Autodesk Inventor part; units mm, degrees
(part 4 of 4)
sketch "Sketch11" plane through (0, 10, 0) normal (0, 1, 0) x (1, 0, 0)
  line L0 (-6.9956, -98.5274) -> (-7.1309, -98.4307) construction
  line L1 (97.89, -8.7381) -> (95.2599, -7.1233) construction
  line L2 (96.5749, -9.4923) -> (97.861, -10.2466) construction
  line L3 (92.9585, -8.419) -> (92.2333, -8.0129) construction
  line L4 (92.5717, -7.1523) -> (92.6491, -7.278) construction
  line L5 (92.6491, -7.278) -> (95.2115, -8.7188) construction
  line L6 (95.724, -6.4464) -> (97.861, -7.7131) construction
  circle A0 centre (0, -95) radius 2 construction
  circle A1 centre (95, 0) radius 2 construction
  line L7 (34.0692, -36.9904) -> (16.7487, -26.9904) construction
  arc A2 (16.7487, -26.9904) -> (16.0167, -24.2583) centre (15.0167, -25.9904) ccw construction
  line L8 (16.0167, -24.2583) -> (29.0167, -1.7417) construction
  arc A3 (29.0167, -1.7417) -> (31.7487, -1.0096) centre (30.0167, -0.0096) ccw construction
  line L9 (31.7487, -1.0096) -> (49.0692, -11.0096) construction
  arc A4 (49.0692, -11.0096) -> (49.8013, -13.7417) centre (50.8013, -12.0096) ccw construction
  line L10 (49.8013, -13.7417) -> (36.8013, -36.2583) construction
  arc A5 (36.8013, -36.2583) -> (34.0692, -36.9904) centre (35.8013, -37.9904) ccw construction
  line L11 (16.0167, -27.7224) -> (33.8013, -37.9904) construction
  arc A6 (33.8013, -37.9904) -> (37.5333, -36.9904) centre (35.8013, -37.9904) ccw construction
  line L12 (37.5333, -36.9904) -> (50.8013, -14.0096) construction
  arc A7 (50.8013, -14.0096) -> (49.8013, -10.2776) centre (50.8013, -12.0096) ccw construction
  line L13 (49.8013, -10.2776) -> (32.0167, -0.0096) construction
  arc A8 (32.0167, -0.0096) -> (28.2846, -1.0096) centre (30.0167, -0.0096) ccw construction
  line L14 (28.2846, -1.0096) -> (15.0167, -23.9904) construction
  arc A9 (15.0167, -23.9904) -> (16.0167, -27.7224) centre (15.0167, -25.9904) ccw construction
  line L15 (-49.0692, -11.0096) -> (-31.7487, -1.0096) construction
  arc A10 (-31.7487, -1.0096) -> (-29.0167, -1.7417) centre (-30.0167, -0.0096) ccw construction
  line L16 (-29.0167, -1.7417) -> (-16.0167, -24.2583) construction
  arc A11 (-16.0167, -24.2583) -> (-16.7487, -26.9904) centre (-15.0167, -25.9904) ccw construction
  line L17 (-16.7487, -26.9904) -> (-34.0692, -36.9904) construction
  arc A12 (-34.0692, -36.9904) -> (-36.8013, -36.2583) centre (-35.8013, -37.9904) ccw construction
  line L18 (-36.8013, -36.2583) -> (-49.8013, -13.7417) construction
  arc A13 (-49.8013, -13.7417) -> (-49.0692, -11.0096) centre (-50.8013, -12.0096) ccw construction
  line L19 (-32.0167, -0.0096) -> (-49.8013, -10.2776) construction
  arc A14 (-49.8013, -10.2776) -> (-50.8013, -14.0096) centre (-50.8013, -12.0096) ccw construction
  line L20 (-50.8013, -14.0096) -> (-37.5333, -36.9904) construction
  arc A15 (-37.5333, -36.9904) -> (-33.8013, -37.9904) centre (-35.8013, -37.9904) ccw construction
  line L21 (-33.8013, -37.9904) -> (-16.0167, -27.7224) construction
  arc A16 (-16.0167, -27.7224) -> (-15.0167, -23.9904) centre (-15.0167, -25.9904) ccw construction
  line L22 (-15.0167, -23.9904) -> (-28.2846, -1.0096) construction
  arc A17 (-28.2846, -1.0096) -> (-32.0167, -0.0096) centre (-30.0167, -0.0096) ccw construction
  line L23 (-46.6246, 31.9097) -> (-46.6246, 8.9097) construction
  line L24 (-46.6246, 8.9097) -> (-69.6246, 8.9097) construction
  line L25 (-69.6246, 8.9097) -> (-69.6246, 31.9097) construction
  line L26 (-69.6246, 31.9097) -> (-46.6246, 31.9097) construction
  line L27 (-45.6246, 7.9097) -> (-45.6246, 32.9097) construction
  line L28 (-45.6246, 32.9097) -> (-70.6246, 32.9097) construction
  line L29 (-70.6246, 32.9097) -> (-70.6246, 7.9097) construction
  line L30 (-70.6246, 7.9097) -> (-45.6246, 7.9097) construction
  line L31 (-23.9006, 30.2452) -> (-23.9006, 7.7452) construction
  line L32 (-23.9006, 7.7452) -> (-41.9006, 7.7452) construction
  line L33 (-41.9006, 7.7452) -> (-41.9006, 30.2452) construction
  line L34 (-41.9006, 30.2452) -> (-23.9006, 30.2452) construction
  line L35 (-32.1006, 6.7452) -> (-22.9006, 6.7452) construction
  line L36 (-22.9006, 6.7452) -> (-22.9006, 31.2452) construction
  line L37 (-22.9006, 31.2452) -> (-32.1006, 31.2452) construction
  arc A18 (-32.1006, 31.2452) -> (-33.7006, 31.2452) centre (-32.9006, 31.2452) ccw construction
  line L38 (-33.7006, 31.2452) -> (-42.9006, 31.2452) construction
  line L39 (-42.9006, 31.2452) -> (-42.9006, 6.7452) construction
  line L40 (-42.9006, 6.7452) -> (-33.7006, 6.7452) construction
  arc A19 (-33.7006, 6.7452) -> (-32.1006, 6.7452) centre (-32.9006, 6.7452) ccw construction
  line L41 (15, 48) -> (15, 28) construction
  arc A20 (15, 28) -> (13, 26) centre (15, 26) ccw construction
  line L42 (13, 26) -> (-13, 26) construction
  arc A21 (-13, 26) -> (-15, 28) centre (-15, 26) ccw construction
  line L43 (-15, 28) -> (-15, 48) construction
  arc A22 (-15, 48) -> (-13, 50) centre (-15, 50) ccw construction
  line L44 (-13, 50) -> (13, 50) construction
  arc A23 (13, 50) -> (15, 48) centre (15, 50) ccw construction
  line L45 (16, 27.7321) -> (16, 48.2679) construction
  arc A24 (16, 48.2679) -> (13.2679, 51) centre (15, 50) ccw construction
  line L46 (13.2679, 51) -> (-13.2679, 51) construction
  arc A25 (-13.2679, 51) -> (-16, 48.2679) centre (-15, 50) ccw construction
  line L47 (-16, 48.2679) -> (-16, 27.7321) construction
  arc A26 (-16, 27.7321) -> (-13.2679, 25) centre (-15, 26) ccw construction
  line L48 (-13.2679, 25) -> (13.2679, 25) construction
  arc A27 (13.2679, 25) -> (16, 27.7321) centre (15, 26) ccw construction
  line L49 (38.8707, 50.1548) -> (54.6756, 59.2798) construction
  line L50 (54.6756, 59.2798) -> (78.6756, 17.7106) construction
  line L51 (78.6756, 17.7106) -> (62.8707, 8.5856) construction
  arc A28 (62.8707, 8.5856) -> (61.5716, 7.8356) centre (62.7211, 7.3446) ccw construction
  line L52 (61.5716, 7.8356) -> (45.7667, -1.2894) construction
  line L53 (45.7667, -1.2894) -> (21.7667, 40.2798) construction
  line L54 (21.7667, 40.2798) -> (37.5716, 49.4048) construction
  arc A29 (37.5716, 49.4048) -> (38.8707, 50.1548) centre (37.7211, 50.6458) ccw construction
  line L55 (63.8037, 7.9696) -> (80.0417, 17.3446) construction
  line L56 (80.0417, 17.3446) -> (55.0417, 60.6458) construction
  line L57 (55.0417, 60.6458) -> (38.8037, 51.2708) construction
  arc A30 (38.8037, 51.2708) -> (36.6386, 50.0208) centre (37.7211, 50.6458) ccw construction
  line L58 (36.6386, 50.0208) -> (20.4006, 40.6458) construction
  line L59 (20.4006, 40.6458) -> (45.4006, -2.6554) construction
  line L60 (45.4006, -2.6554) -> (61.6386, 6.7196) construction
  arc A31 (61.6386, 6.7196) -> (63.8037, 7.9696) centre (62.7211, 7.3446) ccw construction
  line L61 (28, -43) -> (28, -89) construction
  line L62 (28, -89) -> (-28, -89) construction
  line L63 (-28, -89) -> (-28, -43) construction
  line L64 (-28, -43) -> (-8, -43) construction
  line L65 (-8, -43) -> (-8, -43.9952) construction
  line L66 (-8, -43.9952) -> (8, -43.9952) construction
  line L67 (8, -43.9952) -> (8, -43) construction
  line L68 (8, -43) -> (28, -43) construction
  line L69 (-27.75, -90) -> (27.75, -90) construction
  arc A32 (27.75, -90) -> (29, -88.75) centre (29, -90) ccw construction
  line L70 (29, -88.75) -> (29, -43.25) construction
  arc A33 (29, -43.25) -> (27.75, -42) centre (29, -42) ccw construction
  line L71 (27.75, -42) -> (8, -42) construction
  line L72 (8, -42) -> (8, -23.9952) construction
  line L73 (8, -23.9952) -> (-8, -23.9952) construction
  line L74 (-8, -23.9952) -> (-8, -42) construction
  line L75 (-8, -42) -> (-27.75, -42) construction
  arc A34 (-27.75, -42) -> (-29, -43.25) centre (-29, -42) ccw construction
  line L76 (-29, -43.25) -> (-29, -88.75) construction
  arc A35 (-29, -88.75) -> (-27.75, -90) centre (-29, -90) ccw construction
  line L77 (0.5057, 40.2674) -> (2.684, 40.2674) construction
  line L78 (2.684, 40.2674) -> (2.684, 41.3663) construction
  line L79 (0.2042, 43.0389) -> (-1.0405, 43.0389) construction
  line L80 (-1.0405, 43.0389) -> (-1.0405, 32.2253) construction
  line L81 (-1.0405, 32.2253) -> (-3.1702, 32.2253) construction
  line L82 (-3.1702, 32.2253) -> (-3.1702, 31) construction
  line L83 (-3.1702, 31) -> (2.684, 31) construction
  line L84 (2.684, 31) -> (2.684, 32.2253) construction
  line L85 (2.684, 32.2253) -> (0.5057, 32.2253) construction
  line L86 (0.5057, 32.2253) -> (0.5057, 40.2674) construction
  line L87 (11.4709, -68.4771) -> (10.6948, -68.4771) construction
  line L88 (10.6948, -68.4771) -> (10.6948, -69.1) construction
  line L89 (10.6948, -69.1) -> (13.0577, -69.1) construction
  line L90 (13.0577, -69.1) -> (13.0577, -68.4771) construction
  line L91 (13.0577, -68.4771) -> (12.2816, -68.4771) construction
  line L92 (12.2816, -68.4771) -> (12.2816, -63.6229) construction
  line L93 (12.2816, -63.6229) -> (13.0577, -63.6229) construction
  line L94 (13.0577, -63.6229) -> (13.0577, -63) construction
  line L95 (13.0577, -63) -> (10.6948, -63) construction
  line L96 (10.6948, -63) -> (10.6948, -63.6229) construction
  line L97 (10.6948, -63.6229) -> (11.4709, -63.6229) construction
  line L98 (11.4709, -63.6229) -> (11.4709, -68.4771) construction
  line L99 (17.4473, -69.1) -> (17.4473, -63) construction
  line L100 (17.4473, -63) -> (16.6366, -63) construction
  line L101 (16.6366, -63) -> (16.6366, -65.2739) construction
  line L102 (16.6366, -65.2739) -> (15.9495, -65.2739) construction
  line L103 (15.9149, -69.1) -> (17.4473, -69.1) construction
  line L104 (16.0829, -65.966) -> (16.6366, -65.966) construction
  line L105 (16.6366, -65.966) -> (16.6366, -68.3981) construction
  line L106 (16.6366, -68.3981) -> (15.9643, -68.3981) construction
  line L107 (-5.2028, -67.8444) -> (-5.2621, -67.8444) construction
  line L108 (-5.2621, -67.8444) -> (-5.2621, -68.8133) construction
  line L109 (-1.4113, -64.3841) -> (-1.352, -64.3841) construction
  line L110 (-1.352, -64.3841) -> (-1.352, -63.3658) construction
  line L111 (21.0806, -69.1) -> (22.6526, -69.1) construction
  line L112 (22.6526, -69.1) -> (22.6526, -63) construction
  line L113 (22.6526, -63) -> (21.8419, -63) construction
  line L114 (21.8419, -63) -> (21.8419, -65.4271) construction
  line L115 (21.8419, -65.4271) -> (20.9125, -65.4271) construction
  line L116 (20.9125, -65.4271) -> (18.9846, -63) construction
  line L117 (18.9846, -63) -> (17.9317, -63) construction
  line L118 (17.9317, -63) -> (20.1018, -65.6545) construction
  line L119 (21.13, -66.1044) -> (21.8419, -66.1044) construction
  line L120 (21.8419, -66.1044) -> (21.8419, -68.3981) construction
  line L121 (21.8419, -68.3981) -> (21.0361, -68.3981) construction
  line L122 (-10.9568, -63) -> (-11.7279, -63) construction
  line L123 (-11.7279, -63) -> (-11.7279, -67.5775) construction
  line L124 (-11.7279, -67.5775) -> (-10.9568, -67.5775) construction
  line L125 (-10.9568, -67.5775) -> (-10.9568, -63) construction
  line L126 (-15.7419, -65.7979) -> (-13.3246, -65.7979) construction
  line L127 (-13.3246, -65.2096) -> (-16.4932, -65.2096) construction
  line L128 (-16.4932, -65.2096) -> (-16.4932, -65.6298) construction
  line L129 (-16.4092, -63.2818) -> (-16.4092, -64.1221) construction
  line L130 (-16.4092, -64.1221) -> (-16.3647, -64.1221) construction
  line L131 (4.9754, -68.0669) -> (4.9754, -66.0006) construction
  line L132 (4.9754, -66.0006) -> (7.0417, -66.0006) construction
  line L133 (7.0417, -66.0006) -> (7.0417, -65.3431) construction
  line L134 (7.0417, -65.3431) -> (4.9754, -65.3431) construction
  line L135 (4.9754, -65.3431) -> (4.9754, -63.2768) construction
  line L136 (4.9754, -63.2768) -> (4.2932, -63.2768) construction
  line L137 (4.2932, -63.2768) -> (4.2932, -65.3431) construction
  line L138 (4.2932, -65.3431) -> (2.2269, -65.3431) construction
  line L139 (2.2269, -65.3431) -> (2.2269, -66.0006) construction
  line L140 (2.2269, -66.0006) -> (4.2932, -66.0006) construction
  line L141 (4.2932, -66.0006) -> (4.2932, -68.0669) construction
  line L142 (4.2932, -68.0669) -> (4.9754, -68.0669) construction
  line L143 (-17.2891, -63) -> (-18.0603, -63) construction
  line L144 (-18.0603, -63) -> (-18.0603, -69.3719) construction
  line L145 (-18.0603, -69.3719) -> (-17.2891, -69.3719) construction
  line L146 (-17.2891, -69.3719) -> (-17.2891, -63) construction
  line L147 (-6.2656, -69.3719) -> (-6.2656, -63) construction
  line L148 (-6.2656, -63) -> (-7.0368, -63) construction
  line L149 (-7.0368, -63) -> (-7.0368, -66.4207) construction
  line L150 (-9.0882, -65.61) -> (-9.0882, -63) construction
  line L151 (-9.0882, -63) -> (-9.8594, -63) construction
  line L152 (-9.8594, -63) -> (-9.8594, -65.9709) construction
  line L153 (-7.0368, -67.0683) -> (-7.0368, -69.3719) construction
  line L154 (-7.0368, -69.3719) -> (-6.2656, -69.3719) construction
  line L155 (-34.4486, 9.7771) -> (-34.4486, 9.2238) construction
  line L156 (-34.4486, 9.2238) -> (-31.4006, 9.2238) construction
  line L157 (-31.4006, 9.2238) -> (-31.4006, 9.6017) construction
  line L158 (-31.4006, 9.6017) -> (-34.0263, 9.6017) construction
  line L159 (-34.0263, 9.6017) -> (-32.2404, 10.3897) construction
  line L160 (-32.2404, 10.3897) -> (-32.2404, 10.6367) construction
  line L161 (-32.2404, 10.6367) -> (-34.0263, 11.432) construction
  line L162 (-34.0263, 11.432) -> (-31.4006, 11.432) construction
  line L163 (-31.4006, 11.432) -> (-31.4006, 11.8371) construction
  line L164 (-31.4006, 11.8371) -> (-34.4486, 11.8371) construction
  line L165 (-34.4486, 11.8371) -> (-34.4486, 11.2739) construction
  line L166 (-34.4486, 11.2739) -> (-32.7517, 10.5379) construction
  line L167 (-32.7517, 10.5379) -> (-34.4486, 9.7771) construction
  line L168 (-11.7823, -68.3387) -> (-11.7823, -69.1395) construction
  line L169 (-11.7823, -69.1395) -> (-10.9073, -69.1395) construction
  line L170 (-10.9073, -69.1395) -> (-10.9073, -68.3387) construction
  line L171 (-10.9073, -68.3387) -> (-11.7823, -68.3387) construction
  line L172 (-31.4006, 14.769) -> (-31.4006, 15.1543) construction
  line L173 (-31.4006, 15.1543) -> (-34.5845, 15.1543) construction
  line L174 (-34.5845, 15.1543) -> (-34.5845, 14.769) construction
  line L175 (-34.5845, 14.769) -> (-31.4006, 14.769) construction
  line L176 (-21.9407, -63.4647) -> (-21.9407, -63) construction
  line L177 (-21.9407, -63) -> (-22.7119, -63) construction
  line L178 (-22.7119, -63) -> (-22.7119, -69.3719) construction
  line L179 (-22.7119, -69.3719) -> (-21.9407, -69.3719) construction
  line L180 (-21.9407, -69.3719) -> (-21.9407, -67.3946) construction
  line L181 (-21.9407, -66.7569) -> (-21.9407, -64.1122) construction
  line L182 (-31.4006, 17.1303) -> (-31.4006, 17.5157) construction
  line L183 (-31.4006, 17.5157) -> (-33.6879, 17.5157) construction
  line L184 (-33.6879, 17.5157) -> (-33.6879, 17.1303) construction
  line L185 (-33.6879, 17.1303) -> (-31.4006, 17.1303) construction
  line L186 (-35.1477, -24.1889) -> (-33.6654, -23.3332) construction
  line L187 (-33.6654, -23.3332) -> (-33.7092, -23.2574) construction
  line L188 (-26.507, -19.4922) -> (-25.0332, -18.6413) construction
  line L189 (-25.0332, -18.6413) -> (-28.7333, -12.2324) construction
  line L190 (-28.7333, -12.2324) -> (-29.9376, -12.9277) construction
  line L191 (-29.9376, -12.9277) -> (-26.9911, -18.0312) construction
  line L192 (-31.8279, 18.4666) -> (-33.1272, 18.4666) construction
  line L193 (-33.4483, 18.4666) -> (-33.6879, 18.4666) construction
  line L194 (-33.6879, 18.4666) -> (-33.6879, 18.0813) construction
  line L195 (-33.6879, 18.0813) -> (-30.5584, 18.0813) construction
  line L196 (-30.5584, 18.0813) -> (-30.5584, 18.4666) construction
  line L197 (-30.5584, 18.4666) -> (-31.5167, 18.4666) construction
  line L198 (-32.3837, 12.793) -> (-33.6879, 12.793) construction
  line L199 (-33.6879, 12.793) -> (-33.6879, 12.4077) construction
  line L200 (-33.6879, 12.4077) -> (-32.2034, 12.4077) construction
  line L201 (-31.6526, 13.818) -> (-31.4006, 13.818) construction
  line L202 (-31.4006, 13.818) -> (-31.4006, 14.2034) construction
  line L203 (-31.4006, 14.2034) -> (-33.6879, 14.2034) construction
  line L204 (-33.6879, 14.2034) -> (-33.6879, 13.818) construction
  line L205 (-33.6879, 13.818) -> (-31.9786, 13.818) construction
  line L206 (-31.4006, 20.4056) -> (-31.4006, 20.7909) construction
  line L207 (-31.4006, 20.7909) -> (-34.5845, 20.7909) construction
  line L208 (-34.5845, 20.7909) -> (-34.5845, 20.4056) construction
  line L209 (-34.5845, 20.4056) -> (-31.4006, 20.4056) construction
  line L210 (-33.3692, 16.13) -> (-33.3692, 16.8389) construction
  line L211 (-33.3692, 16.8389) -> (-33.6879, 16.8389) construction
  line L212 (-33.6879, 16.8389) -> (-33.6879, 16.13) construction
  line L213 (-33.6879, 16.13) -> (-34.3449, 16.13) construction
  line L214 (-34.3449, 16.13) -> (-34.3449, 15.7446) construction
  line L215 (-34.3449, 15.7446) -> (-33.6879, 15.7446) construction
  line L216 (-33.6879, 15.7446) -> (-33.6879, 15.4853) construction
  line L217 (-33.6879, 15.4853) -> (-33.3692, 15.4853) construction
  line L218 (-33.3692, 15.4853) -> (-33.3692, 15.7446) construction
  line L219 (-33.3692, 15.7446) -> (-32.1021, 15.7446) construction
  line L220 (-31.4204, 16.8389) -> (-31.7662, 16.8389) construction
  line L221 (-31.7662, 16.8389) -> (-31.7662, 16.8166) construction
  line L222 (-32.28, 16.13) -> (-33.3692, 16.13) construction
  line L223 (-32.7987, 27.0771) -> (-32.7987, 25.8692) construction
  line L224 (-32.5047, 25.8692) -> (-32.5047, 27.4525) construction
  line L225 (-32.5047, 27.4525) -> (-32.7147, 27.4525) construction
  line L226 (-31.5414, 27.4105) -> (-31.9613, 27.4105) construction
  line L227 (-31.9613, 27.4105) -> (-31.9613, 27.3883) construction
  line L228 (-34.0683, 17.5428) -> (-34.4684, 17.5428) construction
  line L229 (-34.4684, 17.5428) -> (-34.4684, 17.1056) construction
  line L230 (-34.4684, 17.1056) -> (-34.0683, 17.1056) construction
  line L231 (-34.0683, 17.1056) -> (-34.0683, 17.5428) construction
  line L232 (-33.347, 28.2281) -> (-33.6879, 28.2281) construction
  line L233 (-33.6879, 28.2281) -> (-33.6879, 27.8428) construction
  line L234 (-33.6879, 27.8428) -> (-31.4006, 27.8428) construction
  line L235 (-31.4006, 27.8428) -> (-31.4006, 28.2281) construction
  line L236 (-31.4006, 28.2281) -> (-33.0234, 28.2281) construction
  line L237 (-33.2754, 29.0358) -> (-33.2754, 29.0556) construction
  line L238 (-33.2754, 29.0556) -> (-33.6755, 29.0556) construction
  line L239 (-32.5047, 21.5887) -> (-32.5047, 23.172) construction
  line L240 (-32.5047, 23.172) -> (-32.7147, 23.172) construction
  line L241 (-31.5414, 23.13) -> (-31.9613, 23.13) construction
  line L242 (-31.9613, 23.13) -> (-31.9613, 23.1078) construction
  line L243 (-32.7987, 22.7965) -> (-32.7987, 21.5887) construction
  line L244 (-32.8357, 24.3354) -> (-33.6879, 23.7821) construction
  line L245 (-33.6879, 23.7821) -> (-33.6879, 23.3103) construction
  line L246 (-33.6879, 23.3103) -> (-32.5344, 24.0958) construction
  line L247 (-32.5344, 24.0958) -> (-31.4006, 23.3029) construction
  line L248 (-31.4006, 23.3029) -> (-31.4006, 23.7401) construction
  line L249 (-31.4006, 23.7401) -> (-32.2602, 24.3107) construction
  line L250 (-32.2602, 24.3107) -> (-31.4006, 24.8664) construction
  line L251 (-31.4006, 24.8664) -> (-31.4006, 25.3382) construction
  line L252 (-31.4006, 25.3382) -> (-32.5591, 24.5503) construction
  line L253 (-32.5591, 24.5503) -> (-33.6879, 25.3382) construction
  line L254 (-33.6879, 25.3382) -> (-33.6879, 24.901) construction
  line L255 (-33.6879, 24.901) -> (-32.8357, 24.3354) construction
  line L256 (-54.9741, 18.6224) -> (-54.9741, 20.9097) construction
  line L257 (-54.9741, 20.9097) -> (-55.3594, 20.9097) construction
  line L258 (-55.3594, 20.9097) -> (-55.3594, 19.2004) construction
  line L259 (-56.2708, 19.5858) -> (-56.2708, 20.9097) construction
  line L260 (-56.2708, 20.9097) -> (-56.6561, 20.9097) construction
  line L261 (-56.6561, 20.9097) -> (-56.6561, 19.403) construction
  line L262 (-57.5676, 19.5858) -> (-57.5676, 20.9097) construction
  line L263 (-57.5676, 20.9097) -> (-57.9529, 20.9097) construction
  line L264 (-57.9529, 20.9097) -> (-57.9529, 19.403) construction
  line L265 (-55.3594, 18.8744) -> (-55.3594, 18.6224) construction
  line L266 (-55.3594, 18.6224) -> (-54.9741, 18.6224) construction
  line L267 (-52.3188, 18.5533) -> (-52.3509, 18.5533) construction
  line L268 (-52.3509, 18.5533) -> (-52.3509, 18.0642) construction
  line L269 (-52.3509, 20.7022) -> (-52.3509, 20.2181) construction
  line L270 (-52.3509, 20.2181) -> (-52.3213, 20.2181) construction
  line L271 (-58.4938, 20.9097) -> (-58.8792, 20.9097) construction
  line L272 (-58.8792, 20.9097) -> (-58.8792, 19.2004) construction
  line L273 (-59.7906, 19.5858) -> (-59.7906, 20.9097) construction
  line L274 (-59.7906, 20.9097) -> (-60.1759, 20.9097) construction
  line L275 (-60.1759, 20.9097) -> (-60.1759, 19.403) construction
  line L276 (-61.0874, 19.5858) -> (-61.0874, 20.9097) construction
  line L277 (-61.0874, 20.9097) -> (-61.4727, 20.9097) construction
  line L278 (-61.4727, 20.9097) -> (-61.4727, 19.403) construction
  line L279 (-58.8792, 18.8744) -> (-58.8792, 18.6224) construction
  line L280 (-58.8792, 18.6224) -> (-58.4938, 18.6224) construction
  line L281 (-58.4938, 18.6224) -> (-58.4938, 20.9097) construction
  line L282 (-64.6738, 18.6224) -> (-64.2885, 18.6224) construction
  line L283 (-64.2885, 18.6224) -> (-64.2885, 20.9097) construction
  line L284 (-64.2885, 20.9097) -> (-64.6738, 20.9097) construction
  line L285 (-64.6738, 20.9097) -> (-64.6738, 19.2004) construction
  line L286 (-65.6989, 19.6055) -> (-65.6989, 20.9097) construction
  line L287 (-65.6989, 20.9097) -> (-66.0842, 20.9097) construction
  line L288 (-66.0842, 20.9097) -> (-66.0842, 19.4252) construction
  line L289 (-64.6738, 18.8769) -> (-64.6738, 18.6224) construction
  line L290 (-53.8885, 23.6632) -> (-53.9231, 23.6632) construction
  line L291 (-53.9231, 23.6632) -> (-53.9231, 23.1741) construction
  line L292 (-53.9354, 25.8121) -> (-53.9354, 24.4808) construction
  line L293 (-53.9354, 24.4808) -> (-52.8289, 24.4808) construction
  line L294 (-52.8289, 24.4808) -> (-52.8289, 24.8365) construction
  line L295 (-52.8289, 24.8365) -> (-53.5353, 24.8365) construction
  line L296 (-53.5353, 24.8365) -> (-53.5353, 25.6244) construction
  line L297 (-54.7999, 24.0683) -> (-54.7999, 23.7274) construction
  line L298 (-54.7999, 23.7274) -> (-54.4146, 23.7274) construction
  line L299 (-54.4146, 23.7274) -> (-54.4146, 26.0147) construction
  line L300 (-54.4146, 26.0147) -> (-54.7999, 26.0147) construction
  line L301 (-54.7999, 26.0147) -> (-54.7999, 24.3919) construction
  line L302 (-55.6076, 24.1399) -> (-55.6274, 24.1399) construction
  line L303 (-55.6274, 24.1399) -> (-55.6274, 23.7398) construction
  line L304 (-60.9231, 23.7274) -> (-60.5378, 23.7274) construction
  line L305 (-60.5378, 23.7274) -> (-60.5378, 26.0147) construction
  line L306 (-60.5378, 26.0147) -> (-60.9231, 26.0147) construction
  line L307 (-60.9231, 26.0147) -> (-60.9231, 24.3054) construction
  line L308 (-61.9482, 24.7105) -> (-61.9482, 26.0147) construction
  line L309 (-61.9482, 26.0147) -> (-62.3335, 26.0147) construction
  line L310 (-62.3335, 26.0147) -> (-62.3335, 24.5302) construction
  line L311 (-60.9231, 23.9818) -> (-60.9231, 23.7274) construction
  line L312 (-58.5692, 25.0316) -> (-58.5692, 23.7274) construction
  line L313 (-58.5692, 23.7274) -> (-58.1838, 23.7274) construction
  line L314 (-58.1838, 23.7274) -> (-58.1838, 25.2119) construction
  line L315 (-59.5942, 25.7627) -> (-59.5942, 26.0147) construction
  line L316 (-59.5942, 26.0147) -> (-59.9795, 26.0147) construction
  line L317 (-59.9795, 26.0147) -> (-59.9795, 23.7274) construction
  line L318 (-59.9795, 23.7274) -> (-59.5942, 23.7274) construction
  line L319 (-59.5942, 23.7274) -> (-59.5942, 25.4367) construction
  line L320 (49.0315, 22.2607) -> (50.1317, 22.8959) construction
  line L321 (48.4823, 19.0497) -> (49.163, 19.4427) construction
  line L322 (49.163, 19.4427) -> (49.1408, 19.4812) construction
  line L323 (48.3722, 21.8801) -> (48.5007, 21.9542) construction
  line L324 (50.6883, 23.2173) -> (51.1078, 23.4595) construction
  line L325 (51.1078, 23.4595) -> (50.7222, 24.1273) construction
  line L326 (50.7222, 24.1273) -> (48.0123, 22.5628) construction
  line L327 (-64.2477, 25.7825) -> (-64.2477, 26.0147) construction
  line L328 (-64.2477, 26.0147) -> (-64.6331, 26.0147) construction
  line L329 (-64.6331, 26.0147) -> (-64.6331, 22.8308) construction
  line L330 (-64.6331, 22.8308) -> (-64.2477, 22.8308) construction
  line L331 (-64.2477, 22.8308) -> (-64.2477, 23.8188) construction
  line L332 (-64.2477, 24.1374) -> (-64.2477, 25.4589) construction
  line L333 (48.2466, 24.8956) -> (46.3587, 23.8056) construction
  line L334 (46.3587, 23.8056) -> (45.6493, 25.0342) construction
  line L335 (45.6493, 25.0342) -> (45.0971, 24.7154) construction
  line L336 (45.0971, 24.7154) -> (45.8064, 23.4868) construction
  line L337 (45.8064, 23.4868) -> (44.6677, 22.8293) construction
  line L338 (44.6677, 22.8293) -> (45.0533, 22.1615) construction
  line L339 (45.0533, 22.1615) -> (46.192, 22.8189) construction
  line L340 (46.192, 22.8189) -> (46.4515, 22.3694) construction
  line L341 (46.4515, 22.3694) -> (47.0038, 22.6883) construction
  line L342 (47.0038, 22.6883) -> (46.7443, 23.1378) construction
  line L343 (46.7443, 23.1378) -> (48.9404, 24.4057) construction
  line L344 (49.027, 26.9844) -> (48.4277, 26.6383) construction
  line L345 (48.4277, 26.6383) -> (48.4499, 26.5998) construction
  line L346 (48.7342, 15.3707) -> (49.5424, 13.9708) construction
  line L347 (49.5424, 13.9708) -> (54.8251, 17.0208) construction
  line L348 (54.8251, 17.0208) -> (53.9502, 18.5363) construction
  line L349 (50.3906, 17.9196) -> (50.3649, 17.9048) construction
  line L350 (53.4917, 17.9463) -> (53.8204, 17.3769) construction
  line L351 (53.8204, 17.3769) -> (51.8683, 16.2498) construction
  line L352 (51.8683, 16.2498) -> (51.4086, 17.0461) construction
  line L353 (50.8221, 16.7075) -> (51.2818, 15.9112) construction
  line L354 (51.2818, 15.9112) -> (49.7364, 15.019) construction
  line L355 (49.7364, 15.019) -> (49.3483, 15.6911) construction
  line L356 (43.5091, 31.0249) -> (44.7178, 28.9315) construction
  line L357 (45.2272, 29.2257) -> (43.6429, 31.9698) construction
  line L358 (43.6429, 31.9698) -> (43.279, 31.7597) construction
  line L359 (45.3545, 32.8609) -> (44.6267, 32.4408) construction
  line L360 (44.6267, 32.4408) -> (44.649, 32.4022) construction
  line L361 (44.9548, 26.2372) -> (44.2454, 27.4659) construction
  line L362 (44.2454, 27.4659) -> (43.6932, 27.147) construction
  line L363 (43.6932, 27.147) -> (44.4025, 25.9184) construction
  line L364 (44.4025, 25.9184) -> (43.2638, 25.2609) construction
  line L365 (43.2638, 25.2609) -> (43.6494, 24.5931) construction
  line L366 (43.6494, 24.5931) -> (44.7881, 25.2505) construction
  line L367 (44.7881, 25.2505) -> (45.0476, 24.801) construction
  line L368 (45.0476, 24.801) -> (45.5999, 25.1199) construction
  line L369 (45.5999, 25.1199) -> (45.3404, 25.5694) construction
  line L370 (45.3404, 25.5694) -> (47.5365, 26.8373) construction
  line L371 (47.6231, 29.416) -> (47.0238, 29.0699) construction
  line L372 (47.0238, 29.0699) -> (47.046, 29.0314) construction
  line L373 (46.8427, 27.3272) -> (44.9548, 26.2372) construction
  line L374 (41.407, 32.4712) -> (40.8162, 32.1301) construction
  line L375 (40.8162, 32.1301) -> (41.2018, 31.4623) construction
  line L376 (41.2018, 31.4623) -> (45.166, 33.751) construction
  line L377 (45.166, 33.751) -> (44.7804, 34.4188) construction
  line L378 (44.7804, 34.4188) -> (41.9678, 32.795) construction
  line L379 (40.7229, 33.9427) -> (40.7031, 33.977) construction
  line L380 (40.7031, 33.977) -> (40.0096, 33.5766) construction
  line L381 (41.8523, 37.1177) -> (39.5408, 34.3391) construction
  line L382 (39.5408, 34.3391) -> (39.9561, 33.6199) construction
  line L383 (39.9561, 33.6199) -> (42.8972, 37.2358) construction
  line L384 (42.8972, 37.2358) -> (44.9599, 37.4792) construction
  line L385 (44.9599, 37.4792) -> (44.5472, 38.1941) construction
  line L386 (44.5472, 38.1941) -> (37.8922, 37.1945) construction
  line L387 (37.8922, 37.1945) -> (38.2927, 36.501) construction
  line L388 (38.2927, 36.501) -> (41.8523, 37.1177) construction
  circle A36 centre (50.2211, 28.9952) radius 1.25 construction
  circle A37 centre (0, 0) radius 15 construction
  circle A38 centre (0, 0) radius 100 construction
  line L389 (50.8013, -14.0096) -> (37.5333, -36.9904) construction
  line L390 (44.1673, -25.5) -> (67.55, -39) construction
  line L391 (44.1673, -25.5) -> (71.1673, -25.5) construction
  line L392 (71.8801, -41.5) -> (63.2199, -36.5) construction
  line L393 (72.8801, -39.7679) -> (64.2199, -34.7679)
  line L394 (62.2199, -38.2321) -> (70.8801, -43.2321)
  arc A39 (70.8801, -43.2321) -> (72.8801, -39.7679) centre (71.8801, -41.5) ccw
  arc A40 (64.2199, -34.7679) -> (62.2199, -38.2321) centre (63.2199, -36.5) ccw
  dimension "d92" = 27
  dimension "d93" = 30
  dimension "d94" = 5
  dimension "d95" = 4
  constraints: 12 end point, 4 point on circle, 4 tangent, 2 centre point, 2 midpoint, 1 coincident, 1 equal length, 1 horizontal, 1 parallel, 1 perpendicular, 1 point on line, 358 other
  measures "d92" distance of L390.start L390.end
  measures "d93" angle of L390 L391
  measures "d94" distance of point (67.55, -39) L392.end
  measures "d95" diameter of A40
extrude "Extrusion4" cut sketch "Sketch11" against normal through all
pattern_circular "Circular Pattern2" count 3 over 360 about axis through (0, 0, 0) along (0, 1, 0) of "Extrusion4"
sketch "Sketch12" plane through (0, 10, 0) normal (0, 1, 0) x (1, 0, 0)
  circle A0 centre (0, 0) radius 100 projected
  line L0 (0, 0) -> (0, -98.5) construction
  line L1 (0, 0) -> (-17.1043, -97.0036) construction
  line L2 (0, 0) -> (17.1043, -97.0036) construction
  line L3 (0, 0) -> (98.5, 0) construction
  line L4 (0, 0) -> (97.0036, -17.1043) construction
  line L5 (0, 0) -> (97.0036, 17.1043) construction
  arc A1 (17.1043, -97.0036) -> (97.0036, -17.1043) centre (0, 0) ccw
  arc A2 (97.0036, 17.1043) -> (-17.1043, -97.0036) centre (0, 0) ccw
  arc A3 (16.9307, -96.0188) -> (96.0188, -16.9307) centre (0, 0) ccw
  arc A4 (96.0188, 16.9307) -> (-16.9307, -96.0188) centre (0, 0) ccw
  line L6 (17.1043, -97.0036) -> (16.9307, -96.0188)
  line L7 (-17.1043, -97.0036) -> (-16.9307, -96.0188)
  line L8 (97.0036, -17.1043) -> (96.0188, -16.9307)
  line L9 (97.0036, 17.1043) -> (96.0188, 16.9307)
  dimension "d102" = 10
  dimension "d103" = 10
  dimension "d104" = 10
  dimension "d105" = 10
  dimension "d106" = 98.5
  dimension "d107" = 98.5
  dimension "d108" = 17.1044
  dimension "d109" = 98.5
  dimension "d110" = 1
  dimension "d111" = 1
  constraints: 20 end point, 8 point on circle, 4 centre point, 3 collinear, 3 point on line, 1 horizontal, 1 vertical
  measures "d102" angle of L0 L1
  measures "d103" angle of L2 L0
  measures "d104" angle of L4 L3
  measures "d105" angle of L3 L5
  measures "d106" radius of A1
  measures "d107" radius of A2
  measures "d108" distance from line of L3.end L5
  measures "d109" distance from line of L0.end L3
  measures "d110" radial gap between concentric circles of A1 A3
  measures "d111" radial gap between concentric circles of A2 A4
extrude "Extrusion5" cut sketch "Sketch12" against normal blind 1 contours L6 A3 L8 A1 | L9 A4 L7 A2
body "Solid1"
